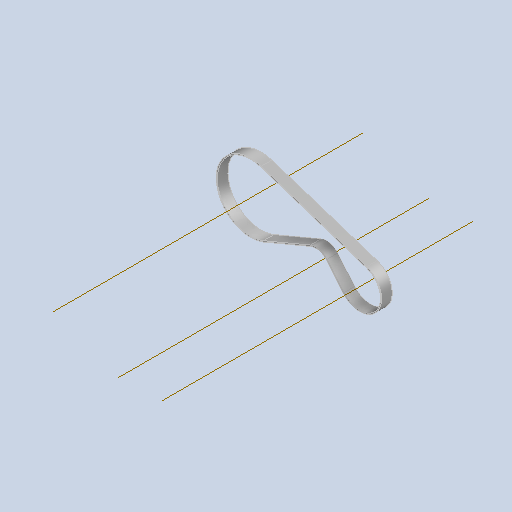
# Autodesk Inventor part: Pas synchroniczny
Saved by Autodesk Inventor 2023 (Build 270158000, 158)
## iProperties
CustomPartVersion: 1
Created: 2023-04-16
Part Number: Pas synchroniczny
Material: Rubber
Document SubType Name: Modeling
Designer: krzys
Density: 0.93 g/cm^3
Appearance: Rubber - Black - Version 1.1
Mass: 3.627 g
Surface Area: 85.8 cm^2
Volume: 3.9 cm^3
Author: krzys
Autodesk Inventor part; units mm, degrees
ref_plane "YZ Plane" through (0, 0, 0) normal (1, 0, 0) x (0, 1, 0)
ref_plane "XZ Plane" through (0, 0, 0) normal (0, 1, 0) x (-1, 0, 0)
ref_plane "XY Plane" through (0, 0, 0) normal (0, 0, 1) x (1, 0, 0)
sketch "Ścieżka szkicu" plane through (0, 0, 0) normal (0, 0, 1) x (1, 0, 0)
  arc A0 (9.8683, 30.2626) -> (12.3244, -29.3483) centre (0, 0) ccw
  arc A1 (87.4874, -33.6895) -> (108.9428, -2.0446) centre (102.7751, -20.9587) ccw
  arc A2 (71.4896, -14.4785) -> (56.4664, -10.8114) centre (61.4998, -22.7975) ccw
  line L0 (56.4664, -10.8114) -> (12.3244, -29.3483)
  line L1 (9.8683, 30.2626) -> (108.9428, -2.0446)
  line L2 (87.4874, -33.6895) -> (71.4896, -14.4785)
  constraints: 6 end point, 6 point on circle, 3 centre point
ref_plane "Płaszczyzna przekroju poprzecznego" through (12.3244, -29.3483, 0) normal (0.9220032, 0.3871822, 0) x (0, 0, 1)
ref_plane "Płaszczyzna konstrukcyjna2" through (0, 0, 0) normal (-1, 0, 0) x (0, 0, 1)
ref_plane "Płaszczyzna konstrukcyjna3" through (102.7751, -20.9587, 0) normal (-0.9382404, 0.3459839, 0) x (0, 0, 1)
sketch "Przekrój poprzeczny" plane through (12.3244, -29.3483, 0) normal (0.9220032, 0.3871822, 0) x (0, 0, 1)
  line L0 (-5, 0.5) -> (5, 0.5)
  line L1 (5, 0.5) -> (5, -0.5)
  line L2 (5, -0.5) -> (-5, -0.5)
  line L3 (-5, -0.5) -> (-5, 0.5)
  line L4 (-5, 0) -> (5, 0) construction
  point P0 (0, 0)
  point P1 (0, 0)
  dimension "d0" = 10
  dimension "d4" = 0.5
  dimension "d5" = 0.5
  constraints: 10 end point, 3 midpoint, 2 parallel, 1 coincident, 1 horizontal, 1 perpendicular, 1 other
  measures "d0" distance between parallel lines of L1 L3
  measures "d4" distance between parallel lines of L2 L4
  measures "d5" distance between parallel lines of L4 L0
sweep "Pas" add profiles "Przekrój poprzeczny" path "Ścieżka szkicu" path curves L2 A2 L0 A0 L1 A1
equation "\"d0\" = da_B"
equation "\"d4\" = da_a"
equation "\"d5\" = da_a2"
equation "\"da_B\" = 10"
equation "\"da_pb\" = 5"
equation "\"da_a\" = 0.5"
equation "\"da_S\" = 2.65"
equation "\"da_Beta\" = 20deg"
equation "\"da_Ht\" = 1.2"
equation "\"da_H\" = 2.2"
equation "\"da_a2\" = 0.5"
body "Solid1"
